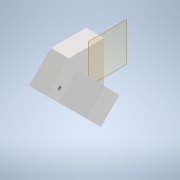
# Autodesk Inventor part: ScrewMount
Saved by Autodesk Inventor 2020 (Build 240168000, 168)
## iProperties
Created: 2015-12-01
Part Number: ScrewMount
Material: Generic
Document SubType Name: Modeling
Designer: physics
Density: 1 g/cm^3
Appearance: Default
Author: physics
Autodesk Inventor part; units mm, degrees
ref_plane "YZ Plane" through (0, 0, 0) normal (1, 0, 0) x (0, 1, 0)
ref_plane "XZ Plane" through (0, 0, 0) normal (0, 1, 0) x (-1, 0, 0)
ref_plane "XY Plane" through (0, 0, 0) normal (0, 0, 1) x (1, 0, 0)
sketch "Sketch1" plane through (0, 0, 0) normal (1, 0, 0) x (0, 1, 0)
  line L0 (0, 0) -> (-40.0558, 0)
  line L1 (-40.0558, 0) -> (-40.0558, -6.35)
  line L2 (-40.0558, -6.35) -> (0, -6.35)
  line L3 (0, -6.35) -> (0, 0)
  line L4 (-23.495, -6.35) -> (-34.0019, 4.1569)
  line L5 (-34.0019, 4.1569) -> (-42.2823, -4.1235)
  line L6 (-42.2823, -4.1235) -> (-31.7754, -14.6304)
  line L7 (-31.7754, -14.6304) -> (-23.495, -6.35)
  line L8 (-23.495, -6.35) -> (-8.636, -6.35) construction
  line L9 (-23.495, -6.35) -> (0, -6.35) construction
  dimension "d0" = 40.0558
  dimension "d2" = 6.35
  dimension "d3" = 14.859
  dimension "d4" = 135
  dimension "d6" = 23.495
  constraints: 20 end point, 4 parallel, 2 horizontal, 2 perpendicular, 2 point on line, 1 collinear, 1 equal length
  measures "d0" distance of L1.end L2.end
  measures "d2" distance of L2.end L0.start
  measures "d3" distance of L4.start L4.end
  measures "d4" angle of L8 L4
  measures "d6" distance of L4.start L2.end
extrude "Extrusion1" add sketch "Sketch1" along normal blind 26.3652
sketch "Sketch2" plane through (26.3652, 0, 0) normal (1, 0, 0) x (0, 0, -1)
  line L0 (6.35, -23.495) -> (6.35, 0) projected
  line L1 (6.35, 0) -> (0, 0) projected
  line L2 (0, 0) -> (0, -29.845) projected
  line L3 (14.6304, -31.7754) -> (6.35, -23.495) projected
  line L4 (6.35, -23.495) -> (0, -29.845)
  line L5 (0, -29.845) -> (0, 0)
  line L6 (0, 0) -> (6.35, 0)
  line L7 (6.35, 0) -> (6.35, -23.495)
  constraints: 8 end point, 3 collinear, 1 perpendicular
extrude "Extrusion2" cut sketch "Sketch2" against normal blind 16.2052
sketch "Sketch5" plane through (0, 0, 0) normal (-1, 0, 0) x (0, 0, 1)
  line L0 (-4.1235, -42.2823) -> (-14.6304, -31.7754) projected
  line L1 (-6.35, -23.495) -> (-6.35, 0) projected
  line L2 (-6.35, -23.495) -> (-6.35, -40.0558)
  line L3 (-6.35, -40.0558) -> (-14.6304, -31.7754)
  line L4 (-14.6304, -31.7754) -> (-6.35, -23.495)
  constraints: 6 end point, 2 collinear, 1 point on line
extrude "Extrusion5" cut sketch "Sketch5" against normal blind 12.7
sketch "Sketch6" plane through (26.3652, -23.495, -6.35) normal (0, 0.7071, -0.7071) x (-1, 0, 0)
  line L0 (13.6652, -11.7103) -> (0, -11.7103) projected
  circle A0 centre (6.8326, -5.8551) radius 4.5085
  line L1 (13.6652, 0) -> (0, 0) projected
  line L2 (0, -11.7103) -> (0, 0) projected
  line L3 (6.8326, -5.8551) -> (6.8326, 0) construction
  line L4 (6.8326, -5.8551) -> (6.8326, -11.7103) construction
  point P0 (26.3652, 21.1036)
  dimension "d24" = 9.017
  constraints: 4 end point, 2 midpoint, 1 centre point, 1 collinear, 1 parallel
  measures "d24" diameter of A0
extrude "Extrusion6" cut sketch "Sketch6" against normal blind 25.4
sketch "Sketch7" plane through (0, 0, 0) normal (-1, 0, 0) x (0, 0, 1)
  line L0 (-6.35, 0) -> (-6.35, -40.0558) projected
  line L1 (-6.35, 0) -> (0, 0) projected
  circle A0 centre (-7.62, -34.9758) radius 2.54
  line L2 (-7.62, -34.9758) -> (-6.35, -34.9758) construction
  line L3 (-6.35, -34.9758) -> (-6.35, -40.0558) construction
  line L4 (-6.35, 0) -> (-6.35, -5.08) construction
  line L5 (-6.35, -5.08) -> (-7.62, -5.08) construction
  circle A1 centre (-7.62, -5.08) radius 2.54
  dimension "d27" = 1.27
  dimension "d29" = 5.08
  dimension "d30" = 5.08
  dimension "d31" = 5.08
  dimension "d32" = 1.27
  dimension "d33" = 5.08
  constraints: 8 end point, 2 centre point, 2 perpendicular, 2 point on line, 1 coincident, 1 collinear
  measures "d27" distance of L2.start L2.end
  measures "d29" diameter of A0
  measures "d30" distance of L2.end L0.end
  measures "d31" diameter of A1
  measures "d32" distance of L4.end L5.end
  measures "d33" distance between parallel lines of L1 L5
extrude "Extrusion7" add sketch "Sketch7" against normal blind 6.35
sketch "Sketch8" plane through (0, 0, 0) normal (-1, 0, 0) x (0, 0, 1)
  line L0 (0, -29.845) -> (4.1569, -34.0019) projected
  line L1 (0, 0) -> (0, -29.845) projected
  line L2 (4.1569, -34.0019) -> (-4.1235, -42.2823) projected
  line L3 (-6.35, -7.2797) -> (-6.35, -32.7761) projected
  line L4 (4.1569, -34.0019) -> (4.1569, -26.3819)
  line L5 (4.1569, -26.3819) -> (0, -22.225)
  line L6 (0, -22.225) -> (0, -29.845)
  line L7 (4.1569, -34.0019) -> (0, -29.845)
  dimension "d42" = 7.62
  constraints: 8 end point, 2 collinear, 1 parallel, 1 perpendicular, 1 point on line
  measures "d42" distance of L5.end L0.start
extrude "Extrusion8" add sketch "Sketch8" against normal blind 12.1412
ref_plane "Work Plane1" through (12.1412, -6.35, -6.35) normal (1, 0, 0) x (0, 0, -1)
sketch "Sketch9" plane through (12.1412, -6.35, -6.35) normal (1, 0, 0) x (0, 0, -1)
  line L0 (-10.5069, 6.35) -> (-10.5069, -29.5569) projected
  line L1 (-6.35, -25.4) -> (-10.5069, -29.5569) projected
  line L2 (-6.35, -25.4) -> (-6.35, 0) projected
  circle A0 centre (-8.4284, -20.4934) radius 1.5875
  line L3 (-6.35, -20.4934) -> (-10.5069, -20.4934) construction
  line L4 (-8.4284, -20.4934) -> (-8.4284, -27.4784) construction
  point P0 (-6.35, 6.35)
  dimension "d38" = 3.175
  dimension "d39" = 6.985
  constraints: 4 end point, 2 midpoint, 2 perpendicular, 2 point on line, 1 centre point, 1 coincident
  measures "d38" diameter of A0
  measures "d39" distance of L4.start L4.end
extrude "Extrusion9" add sketch "Sketch9" along normal blind 2.54
sketch "Sketch10" plane through (26.3652, 0, 0) normal (1, 0, 0) x (0, 0, -1)
  line L0 (0, -40.0558) -> (1.897, -40.0558) projected
  line L1 (14.6304, -31.7754) -> (6.35, -23.495) projected
  line L2 (0, -38.1254) -> (1.897, -40.0558)
  line L3 (1.897, -40.0558) -> (0, -40.0558)
  line L4 (0, -38.1254) -> (0, -40.0558)
  line L5 (0, -38.1254) -> (1.897, -40.0558)
  point P0 (0, 0)
  dimension "d43" = 0.5
  constraints: 8 end point, 2 collinear, 1 perpendicular
  measures "d43" angle of L1 L2
extrude "Extrusion10" cut sketch "Sketch10" against normal blind 38.1
sketch "Sketch11" plane through (14.6812, -26.8434, 2.0784) normal (1, 0, 0) x (0, 0, -1)
  circle A0 centre (0, 0) radius 1.5875 projected
  circle A1 centre (0, 0) radius 1.5875
  line L0 (-1.5875, 0) -> (1.5875, 0)
  line L1 (1.5875, 0) -> (1.5875, -2.159)
  line L2 (1.5875, -2.159) -> (-1.5875, -2.159)
  line L3 (-1.5875, -2.159) -> (-1.5875, 0)
  point P0 (2.0784, 26.8434)
  dimension "d46" = 2.159
  constraints: 8 end point, 2 horizontal, 2 horizontal alignment, 2 parallel, 1 coincident, 1 perpendicular, 1 vertical, 3 other
  measures "d46" distance of L0.end L1.end
extrude "Extrusion11" add sketch "Sketch11" along normal blind 2.54
sketch "Sketch14" plane through (12.1412, -6.35, -6.35) normal (1, 0, 0) x (0, 0, -1)
  line L0 (-6.8465, -10.2985) -> (-15.1263, -2.0187)
  line L1 (8.2804, -25.4254) -> (0, -17.145) projected
  line L2 (-15.1263, -2.0187) -> (-25.6332, -12.5256)
  line L3 (-25.6332, -12.5256) -> (-17.3534, -20.8054)
  line L4 (-17.3534, -20.8054) -> (-6.8465, -10.2985)
  point P0 (-6.35, 6.35)
  dimension "d60" = 11.7094
  dimension "d61" = 14.859
  constraints: 8 end point, 2 perpendicular, 1 collinear, 1 parallel
  measures "d60" distance of L0.start L0.end
  measures "d61" distance of L0.end L2.end
extrude "Extrusion14" add sketch "Sketch14" along normal blind 13.6652
sketch "Sketch15" plane through (12.1412, -6.35, -6.35) normal (-1, 0, 0) x (0, 0, 1)
  line L0 (6.8465, -10.2985) -> (15.1263, -2.0187) projected
  line L1 (25.6332, -12.5256) -> (17.3534, -20.8054) projected
  line L2 (15.1263, -2.0187) -> (25.6332, -12.5256)
  line L3 (25.6332, -12.5256) -> (17.3534, -20.8054)
  line L4 (6.8465, -10.2985) -> (17.3534, -20.8054)
  line L5 (6.8465, -10.2985) -> (15.1263, -2.0187)
  point P0 (6.35, 6.35)
  constraints: 8 end point, 2 perpendicular, 1 collinear
extrude "Extrusion15" add sketch "Sketch15" along normal up to surface (12.1412 mm away)
sketch "Sketch17" plane through (0, 0, 0) normal (-1, 0, 0) x (0, 0, 1)
  line L0 (-1.897, -40.0558) -> (0, -38.1254) projected
  line L1 (4.1569, -26.3819) -> (0, -22.225) projected
  line L2 (0, 0) -> (0, -22.225) projected
  line L3 (-6.35, -37.1755) -> (-6.35, -40.0558) projected
  line L4 (-1.897, -40.0558) -> (-4.1235, -42.2823) projected
  line L5 (0, 0) -> (0, -22.225)
  line L6 (0, -22.225) -> (3.1163, -19.1087)
  line L7 (3.1163, -19.1087) -> (11.1874, -11.0376)
  line L8 (11.1874, -11.0376) -> (8.66, -8.5101)
  line L9 (8.66, -8.5101) -> (0, 0)
  constraints: 10 end point, 2 parallel, 2 perpendicular, 1 collinear, 1 point on line
extrude "Extrusion17" add sketch "Sketch17" against normal up to surface (10.16 mm away)
sketch "Sketch18" plane through (25.8064, -8.3687, 8.7763) normal (0, 0.7071, -0.7071) x (-1, 0, 0)
  circle A0 centre (6.5407, -5.8547) radius 4.5085
  point P0 (25.8064, -0.2882)
  dimension "d70" = 9.017
  constraints: 1 centre point
  measures "d70" diameter of A0
extrude "Extrusion18" cut sketch "Sketch18" against normal up to surface (14.859 mm away)
sketch "Sketch19" plane through (26.3652, 0, 0) normal (1, 0, 0) x (0, 0, -1)
  line L0 (0, -38.1588) -> (0, -38.1254) projected
  line L1 (0, -38.1254) -> (1.897, -40.0558) projected
  line L2 (1.897, -40.0558) -> (4.1235, -42.2823) projected
  line L3 (14.6304, -31.7754) -> (6.35, -23.495) projected
  line L4 (-4.1569, -34.0019) -> (0, -38.1588) projected
  line L5 (-4.1569, -34.0019) -> (6.35, -23.495)
  line L6 (14.6304, -31.7754) -> (6.35, -23.495)
  line L7 (14.6304, -31.7754) -> (4.1235, -42.2823)
  line L8 (-4.1569, -34.0019) -> (4.1235, -42.2823)
  point P0 (0, 0)
  constraints: 8 end point, 1 collinear, 1 perpendicular
extrude "Extrusion19" cut sketch "Sketch19" against normal up to surface (16.2052 mm away) contours L4 L5 L3 L7 L2 L1 L0
sketch "Sketch21" plane through (10.16, 0, 0) normal (1, 0, 0) x (0, 0, -1)
  line L0 (-8.6473, -8.4977) -> (0, 0) projected
  line L1 (0, 0) -> (-19.2606, -18.9274)
  line L2 (-19.2606, -18.9274) -> (-25.9368, -12.1336)
  line L3 (0, 0) -> (-6.6762, 6.7937)
  line L4 (-6.6762, 6.7937) -> (-25.9368, -12.1336)
  line L5 (0, 0) -> (-4.5719, 0)
  line L6 (-4.5719, 0) -> (-13.5895, 0)
  dimension "d75" = 9.525
  constraints: 12 end point, 2 perpendicular, 2 point on line, 1 collinear
  measures "d75" distance of L1.end L2.end
extrude "Extrusion21" add sketch "Sketch21" against normal up to surface (10.16 mm away) contours L1 L2 L4 L6 L5 L0
sketch "Sketch22" plane through (10.16, 0, 0) normal (1, 0, 0) x (0, 0, -1)
  line L0 (-8.7763, -8.3687) -> (-19.2832, -18.8756) projected
  circle A0 centre (-18.8774, -12.1837) radius 1.588
  line L1 (-25.9368, -12.1336) -> (-19.2606, -18.9274) projected
  point P0 (0, 0)
  dimension "d81" = 3.176
  dimension "d82" = 4.445
  dimension "d95" = 5
  constraints: 1 centre point
  measures "d81" diameter of A0
  measures "d82" distance from line of L0 A0.centre
  measures "d95" distance from line of L1 A0.centre
extrude "Extrusion22" [suppressed]
sketch "Sketch23" plane through (24.2316, -12.1837, 18.8774) normal (1, 0, 0) x (0, 0, -1)
  circle A0 centre (0, 0) radius 1.588 projected
  circle A1 centre (0, 0) radius 1.588
  line L0 (0.0027, 1.588) -> (-2.1563, 1.588)
  line L1 (-2.1563, 1.588) -> (-2.1563, -1.588)
  line L2 (-2.1563, -1.588) -> (0.0027, -1.588)
  line L3 (0.0027, -1.588) -> (0.0027, 1.588)
  point P0 (18.8774, 12.1837)
  dimension "d85" = 2.159
  constraints: 8 end point, 2 parallel, 1 coincident, 1 horizontal, 1 perpendicular, 5 other
  measures "d85" distance of L2.end L1.end
extrude "Extrusion23" [suppressed]
sketch "Sketch24" plane through (10.16, 0, 0) normal (1, 0, 0) x (0, 0, -1)
  line L0 (6.35, 0) -> (6.35, -40.0558) projected
  line L1 (-13.5895, 0) -> (6.35, 0) projected
  line L2 (-13.5895, 0) -> (-25.9368, -12.1336) projected
  line L3 (-25.9368, -12.1336) -> (-19.2606, -18.9274) projected
  line L4 (-19.2606, -18.9274) -> (-19.2459, -18.9129) projected
  line L5 (-19.2832, -18.8756) -> (-19.2459, -18.9129) projected
  line L6 (-8.7763, -8.3687) -> (-19.2832, -18.8756) projected
  line L7 (-0.4965, -16.6485) -> (-8.7763, -8.3687) projected
  line L8 (-3.0365, -19.1885) -> (-0.4965, -16.6485) projected
  line L9 (0, -22.225) -> (-3.0365, -19.1885) projected
  line L10 (0, -29.845) -> (0, -22.225) projected
  line L11 (-4.1569, -34.0019) -> (0, -29.845) projected
  line L12 (0, -38.1588) -> (-4.1569, -34.0019) projected
  line L13 (0, -38.1254) -> (0, -38.1588) projected
  line L14 (1.897, -40.0558) -> (0, -38.1254) projected
  line L15 (4.1235, -42.2823) -> (1.897, -40.0558) projected
  line L16 (6.35, -40.0558) -> (4.1235, -42.2823) projected
  line L17 (-4.1569, -34.0019) -> (0, -34.0019)
  line L18 (0, -34.0019) -> (0, -22.225)
  line L19 (0, -22.225) -> (-4.1569, -22.225)
  line L20 (-4.1569, -22.225) -> (-4.1569, -34.0019)
  point P0 (0, 0)
  constraints: 8 end point, 2 parallel, 1 horizontal, 1 perpendicular
extrude "Extrusion24" cut sketch "Sketch24" along normal up to surface (7.0612 mm away) contours L20 L19 L10 L11 | L11 L18 L17
sketch "Sketch25" plane through (10.16, 0, 0) normal (1, 0, 0) x (0, 0, -1)
  line L0 (-4.1569, -34.0019) -> (-4.1569, -26.3819) projected
  line L1 (-4.1569, -34.0019) -> (-4.1569, -26.3819)
  line L2 (-4.1569, -26.3819) -> (0, -22.225)
  line L3 (0, -22.225) -> (-3.0365, -19.1885)
  line L4 (-4.1569, -34.0019) -> (-11.3495, -26.8093)
  line L5 (-11.3495, -26.8093) -> (-3.0365, -19.1885)
  point P0 (0, 0)
  constraints: 10 end point, 1 collinear, 1 parallel
extrude "Extrusion25" add sketch "Sketch25" against normal up to surface (10.16 mm away)
sketch "Sketch26" plane through (10.16, 0, 0) normal (1, 0, 0) x (0, 0, -1)
  circle A0 centre (-18.8774, -12.1837) radius 1.588 projected
  circle A1 centre (-18.8774, -12.1837) radius 2.54
  point P0 (0, 0)
  dimension "d92" = 5.08
  constraints: 1 centre point, 1 coincident
  measures "d92" diameter of A1
extrude "Extrusion26" [suppressed]
sketch "Sketch27" plane through (10.16, 0, 0) normal (1, 0, 0) x (0, 0, -1)
  circle A0 centre (-18.8774, -12.1837) radius 1.588 projected
  line L0 (-25.9368, -12.1336) -> (-19.2606, -18.9274) projected
  line L1 (-13.5895, 0) -> (-25.9368, -12.1336) projected
  point P0 (0, 0)
  dimension "d96" = 5
  dimension "d97" = 4.9837
  constraints: 1 coincident
  measures "d96" distance from line of L0 A0.centre
  measures "d97" distance from line of A0.centre L1
hole "Hole1" at (10.16, -12.1837, 18.8774) direction (-1, 0, 0) diameter 2.1565 end through all thread size "4-40 UNC" class "2B" standard "ANSI Unified Screw Threads"
body "Solid1"
